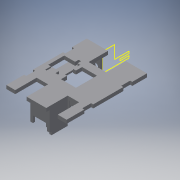
# Autodesk Inventor part: Fronthalf1
Saved by Autodesk Inventor 2016 (Build 200138000, 138)
## iProperties
Created: 2017-03-04
Part Number: Fronthalf1
Material: Generic
Document SubType Name: Modeling
Designer: Owner
Density: 1 g/cm^3
Appearance: Default
Author: Owner
Autodesk Inventor part; units mm, degrees
ref_plane "YZ Plane" through (0, 0, 0) normal (1, 0, 0) x (0, 1, 0)
ref_plane "XZ Plane" through (0, 0, 0) normal (0, 1, 0) x (-1, 0, 0)
ref_plane "XY Plane" through (0, 0, 0) normal (0, 0, 1) x (1, 0, 0)
sketch "Sketch1" plane through (0, 0, 0) normal (0, 1, 0) x (-1, 0, 0)
  line L0 (0, 0) -> (0, 114.3)
  line L1 (0, 114.3) -> (76.2, 114.3)
  line L2 (76.2, 114.3) -> (76.2, 0)
  line L3 (76.2, 0) -> (0, 0)
  circle A0 centre (38.1, 0) radius 38.1
  dimension "d0" = 114.3
  dimension "d1" = 76.2
  constraints: 8 end point, 2 perpendicular, 2 vertical, 1 horizontal alignment, 1 midpoint, 2 other
  measures "d0" distance of L0.start L0.end
  measures "d1" distance of L0.end L1.end
extrude "Extrusion1" add sketch "Sketch1" along normal blind 5
sketch "Sketch2" plane through (0, 0, 0) normal (0, -1, 0) x (1, 0, 0)
  line L0 (-27.94, 89.7) -> (-27.94, 77) projected
  line L1 (-48.26, 51.6) -> (-48.26, 64.3) projected
  line L2 (-48.26, 51.6) -> (-48.26, 49.6)
  line L3 (-53.34, 64.3) -> (-48.26, 64.3)
  line L4 (-48.26, 64.3) -> (-48.26, 66.3)
  line L5 (-27.94, 66.3) -> (-27.94, 49.6)
  line L6 (-48.26, 70.015) -> (-48.26, 45.885) projected
  line L7 (-48.26, 70.015) -> (-48.26, 45.885)
  line L8 (-48.26, 42.885) -> (-27.94, 42.885)
  line L9 (-27.94, 42.885) -> (-27.94, 72.015)
  line L10 (-27.94, 72.015) -> (-27.94, 73.015)
  line L11 (-27.94, 73.015) -> (-48.26, 73.015)
  line L12 (-48.26, 42.885) -> (-49.26, 42.885)
  line L13 (-49.0223, 73.0219) -> (-48.26, 73.015)
  line L14 (-27.94, 73.015) -> (-49.26, 73.015)
  line L15 (-49.26, 73.015) -> (-49.26, 42.885)
  line L16 (-49.26, 42.885) -> (-27.94, 42.885)
  line L17 (-27.94, 42.885) -> (-27.94, 73.015)
  point P0 (0, 0)
  dimension "d5" = 2
  dimension "d12" = 2
  dimension "d69" = 3
  dimension "d70" = 3
  dimension "d75" = 1
  constraints: 30 end point, 3 equal length, 3 horizontal, 3 perpendicular, 2 point on line, 2 vertical, 1 other
  measures "d5" distance of L1.start L2.end
  measures "d12" distance of L1.end L4.end
  measures "d69" distance of L6.start L11.end
  measures "d70" distance of L6.end L8.start
  measures "d75" distance of L8.start L12.end
extrude "Extrusion2" cut sketch "Sketch2" against normal blind 25.4
sketch "Sketch3" plane through (0, 0, 0) normal (0, -1, 0) x (1, 0, 0)
  arc A0 (-76.2, 0) -> (0, 0) centre (-38.1, 0) ccw projected
  line L0 (-38.1, 0) -> (-38.1, -27.5)
  circle A1 centre (-38.1, -27.5) radius 5
  dimension "d8" = 27.5
  dimension "d9" = 10
  constraints: 2 end point, 1 centre point, 1 coincident, 1 vertical
  measures "d8" distance of L0.start L0.end
  measures "d9" diameter of A1
extrude "Extrusion3" cut sketch "Sketch3" against normal blind 25.4
sketch "Sketch5" plane through (-76.2, 0, 114.3) normal (0, 0, 1) x (1, 0, 0)
  circle A0 centre (38.1, -23.375) radius 3.275 projected
  line L0 (47.85, -18.65) -> (28.35, -18.65) projected
  line L1 (28.35, -28.1) -> (47.85, -28.1) projected
  line L2 (28.35, -18.65) -> (28.35, -28.1) projected
  line L3 (47.85, -28.1) -> (47.85, -18.65) projected
  line L4 (76.2, 5) -> (0, 5) projected
  line L5 (38.1, 5) -> (38.1, -18.65)
  line L6 (38.1, -18.65) -> (47.85, -18.65)
  line L7 (47.85, -18.65) -> (48.1, -18.65)
  line L8 (48.1, -18.65) -> (48.1, -28.1)
  line L9 (48.1, -28.1) -> (52.1, -28.1)
  line L10 (52.1, -28.1) -> (52.1, -18.65)
  line L11 (52.1, -18.65) -> (52.1, -16.65)
  line L12 (52.1, -16.65) -> (52.1, 0)
  line L13 (0, 0) -> (76.2, 0) projected
  line L14 (38.1, -18.65) -> (28.35, -18.65)
  line L15 (28.35, -18.65) -> (28.1, -18.65)
  line L16 (28.1, -18.65) -> (28.1, -28.1)
  line L17 (28.1, -28.1) -> (24.1, -28.1)
  line L18 (24.1, -28.1) -> (24.1, 0)
  line L19 (52.1, 0) -> (24.1, 0)
  dimension "d23" = 0.25
  dimension "d24" = 4
  dimension "d25" = 2
  dimension "d26" = 0.25
  dimension "d27" = 4
  constraints: 28 end point, 9 point on line, 7 perpendicular, 2 midpoint, 1 collinear
  measures "d23" distance of L0.start L7.end
  measures "d24" distance of L8.end L9.end
  measures "d25" distance of L10.end L11.end
  measures "d26" distance of L0.end L15.end
  measures "d27" distance of L16.end L17.end
extrude "Extrusion5" add sketch "Sketch5" against normal blind 3 contours L0 L5 L13 L12 L11 L10 L9 L8 L7 | L0 L15 L16 L17 L18 L13 L5
ref_plane "Work Plane1" through (-76.2, 0, 79.55) normal (0, 0, -1) x (-1, 0, 0)
sketch "Sketch6" plane through (-76.2, 0, 79.55) normal (0, 0, -1) x (-1, 0, 0)
  circle A0 centre (-38.1, -23.375) radius 3.275 projected
  line L0 (-34.825, -23.375) -> (-30.825, -23.375)
  line L1 (-48.1, -18.65) -> (-28.1, -18.65) projected
  line L2 (-30.825, -23.375) -> (-30.825, 0)
  line L3 (-41.375, -23.375) -> (-45.375, -23.375)
  line L4 (0, 5) -> (-76.2, 5) projected
  line L5 (-45.375, -23.375) -> (-45.375, 0)
  line L6 (-45.375, 0) -> (-30.825, 0)
  circle A1 centre (-38.1, -23.375) radius 3.275
  point P0 (-76.2, 0)
  dimension "d31" = 4
  dimension "d32" = 4
  constraints: 10 end point, 3 perpendicular, 2 parallel, 2 point on circle, 1 centre point, 1 coincident, 1 concentric
  measures "d31" distance of L0.start L0.end
  measures "d32" distance of L3.start L3.end
extrude "Extrusion6" add sketch "Sketch6" along normal blind 3 contours A0 L3 L5 L1 L2 L0 | L1 L5 L6 L2
sketch "Sketch9" plane through (0, 0, 0) normal (0, -1, 0) x (1, 0, 0)
  line L0 (-45.375, 79.55) -> (-45.375, 76.55) projected
  line L1 (-44.442, 86.368) -> (-46.442, 86.368) projected
  line L2 (-46.442, 86.368) -> (-46.442, 79.796) projected
  line L3 (-46.442, 79.796) -> (-38.902, 79.796) projected
  line L4 (-38.902, 79.796) -> (-38.902, 86.368) projected
  line L5 (-38.902, 86.368) -> (-40.902, 86.368) projected
  line L6 (-40.902, 86.368) -> (-40.902, 81.796) projected
  line L7 (-40.902, 81.796) -> (-44.442, 81.796) projected
  line L8 (-44.442, 81.796) -> (-44.442, 86.368) projected
  line L9 (-41.375, 79.55) -> (-45.375, 79.55) projected
  line L10 (-45.375, 79.55) -> (-45.375, 76.55) projected
  line L11 (-41.375, 76.55) -> (-45.375, 76.55) projected
  line L12 (-41.375, 79.55) -> (-41.375, 76.55) projected
  line L13 (-45.375, 76.55) -> (-45.375, 79.55) projected
  line L14 (-46.442, 79.796) -> (-45.375, 79.796)
  line L15 (-45.375, 79.796) -> (-45.375, 76.55)
  line L16 (-45.375, 76.55) -> (-46.442, 76.55)
  line L17 (-46.442, 76.55) -> (-46.442, 79.796)
  line L18 (-38.902, 86.368) -> (-38.902, 79.796) projected
  line L19 (-38.902, 79.796) -> (-45.375, 79.796)
  line L20 (-45.375, 79.796) -> (-45.375, 79.55)
  line L21 (-45.375, 79.55) -> (-38.902, 79.55)
  line L22 (-38.902, 79.55) -> (-38.902, 79.796)
  point P0 (0, 0)
  constraints: 16 end point, 4 parallel, 2 horizontal, 2 perpendicular
extrude "Extrusion9" add sketch "Sketch9" along normal blind 23.37 contours L15 L3 L22 L21 L9 | L0 L16 L17 L3 L15
sketch "Sketch14" plane through (0, 0, 0) normal (0, -1, 0) x (1, 0, 0)
  line L0 (0, 0) -> (5, 0)
  line L1 (5, 0) -> (5, 114.3)
  line L2 (5, 114.3) -> (5, 119.3)
  line L3 (5, 119.3) -> (-76.2, 119.3)
  line L4 (-52.1, 114.3) -> (-76.2, 114.3) projected
  line L5 (-76.2, 119.3) -> (-81.2, 119.3)
  line L6 (-81.2, 119.3) -> (-81.2, 0)
  line L7 (-76.2, 0) -> (-81.2, 0)
  line L8 (-81.2, 0) -> (-81.2, 119.3)
  line L9 (-81.2, 119.3) -> (-76.2, 119.3)
  line L10 (-76.2, 119.3) -> (-76.2, 0)
  line L11 (-81.2, 119.3) -> (5, 119.3)
  line L12 (5, 119.3) -> (5, 114.3)
  line L13 (5, 114.3) -> (-81.2, 114.3)
  line L14 (-81.2, 114.3) -> (-81.2, 119.3)
  line L15 (5, 119.3) -> (0, 119.3)
  line L16 (0, 119.3) -> (0, 0)
  line L17 (0, 0) -> (5, 0)
  line L18 (5, 0) -> (5, 119.3)
  dimension "d58" = 5
  dimension "d59" = 5
  dimension "d60" = 5
  constraints: 36 end point, 7 parallel, 5 perpendicular, 4 horizontal, 3 point on line
  measures "d58" distance of L0.start L0.end
  measures "d59" distance of L1.end L2.end
  measures "d60" distance of L3.end L5.end
extrude "Extrusion14" add sketch "Sketch14" against normal blind 5
sketch "Sketch15" plane through (-38.902, -23.37, 79.55) normal (0, 0, -1) x (-1, 0, 0)
  arc A0 (2.473, -0.005) -> (-4.077, -0.005) centre (-0.802, -0.005) ccw projected
  circle A1 centre (-0.802, -0.005) radius 3.275
  point P0 (-38.902, 23.37)
  constraints: 1 centre point, 1 coincident
extrude "Extrusion15" cut sketch "Sketch15" against normal blind 25.4
ref_plane "Work Plane2" through (-29.1001, -34.45, 98.298) normal (1, 0, 0) x (0, -1, 0)
sketch "Sketch16" plane through (-29.1001, -34.45, 98.298) normal (1, 0, 0) x (0, -1, 0)
  line L0 (-5.08, 11.43) -> (5.08, 11.43) projected
  arc A0 (-5.08, 11.43) -> (-6.35, 10.16) centre (-5.08, 10.16) ccw projected
  line L1 (-6.35, -10.16) -> (-6.35, 10.16) projected
  arc A1 (-6.35, -10.16) -> (-5.08, -11.43) centre (-5.08, -10.16) ccw projected
  line L2 (5.08, -11.43) -> (-5.08, -11.43) projected
  arc A2 (5.08, -11.43) -> (6.35, -10.16) centre (5.08, -10.16) ccw projected
  line L3 (6.35, 10.16) -> (6.35, -10.16) projected
  arc A3 (6.35, 10.16) -> (5.08, 11.43) centre (5.08, 10.16) ccw projected
  line L4 (0, 11.43) -> (-6.35, 11.43)
  line L5 (-6.35, 11.43) -> (-6.35, -11.43)
  line L6 (-6.35, -11.43) -> (0, -11.43)
  line L7 (0, -11.43) -> (0, 11.43)
  line L8 (-34.45, -21.002) -> (-34.45, 98.298) projected
  line L9 (-6.35, 11.43) -> (-34.45, 11.43)
  line L10 (-34.45, 11.43) -> (-34.45, -11.43)
  line L11 (-34.45, -11.43) -> (-6.35, -11.43)
  line L12 (-6.35, -11.43) -> (-6.35, 11.43)
  constraints: 16 end point, 4 parallel, 2 horizontal, 2 perpendicular, 2 point on line, 1 midpoint
extrude "Extrusion16" add sketch "Sketch16" along normal blind 3 contours L0 L7 L2 A1 L1 A0 | A0 L5 L4 | L1 L5 L11 L8 L9 | A1 L6 L5
sketch "Sketch17" plane through (-29.1001, -34.45, 98.298) normal (-1, 0, 0) x (0, 0, 1)
  line L0 (10.16, 6.35) -> (-10.16, 6.35) projected
  line L1 (11.43, 34.45) -> (11.43, 0) projected
  line L2 (11.43, 34.45) -> (-11.43, 34.45) projected
  line L3 (11.43, 6.35) -> (-11.43, 6.35)
  line L4 (-11.43, 6.35) -> (-11.43, 34.45)
  line L5 (-11.43, 34.45) -> (11.43, 34.45)
  line L6 (11.43, 34.45) -> (11.43, 6.35)
  point P0 (-98.298, 34.45)
  constraints: 8 end point, 2 parallel, 1 horizontal, 1 perpendicular, 1 point on line
extrude "Extrusion17" add sketch "Sketch17" along normal blind 5
sketch "Sketch18" plane through (0, 0, 0) normal (0, -1, 0) x (1, 0, 0)
  line L0 (-76.2, 64.3) -> (-60.198, 64.3) projected
  line L1 (-70.866, 64.3) -> (-71.882, 64.3) projected
  line L2 (-70.866, 64.3) -> (-70.866, 66.84) projected
  line L3 (-71.882, 66.84) -> (-70.866, 66.84) projected
  line L4 (-76.2, 63.03) -> (-76.2, 64.3) projected
  line L5 (-76.2, 63.03) -> (-76.2, 42.71) projected
  line L6 (-76.2, 41.44) -> (-76.2, 42.71) projected
  line L7 (-76.2, 41.44) -> (-60.198, 41.44) projected
  line L8 (-60.198, 36.868) -> (-60.198, 42.71) projected
  line L9 (-57.658, 36.868) -> (-60.198, 36.868) projected
  line L10 (-57.658, 36.868) -> (-57.658, 42.71) projected
  line L11 (-57.658, 41.44) -> (-53.34, 41.44) projected
  line L12 (-53.34, 57.95) -> (-53.34, 42.71) projected
  line L13 (-53.34, 41.44) -> (-53.34, 42.71) projected
  line L14 (-53.34, 51.6) -> (-48.26, 51.6)
  line L15 (-53.34, 64.3) -> (-48.26, 64.3)
  line L16 (-57.658, 64.3) -> (-53.34, 64.3) projected
  line L17 (-57.658, 63.03) -> (-57.658, 68.872) projected
  line L18 (-60.198, 63.03) -> (-60.198, 68.872) projected
  line L19 (-57.658, 68.872) -> (-60.198, 68.872) projected
  line L20 (-48.26, 70.015) -> (-48.26, 45.885) projected
  line L21 (-76.2, 64.3) -> (-53.34, 64.3)
  line L22 (-53.34, 64.3) -> (-53.34, 41.44)
  line L23 (-53.34, 41.44) -> (-76.2, 41.44)
  line L24 (-76.2, 41.44) -> (-76.2, 64.3)
  line L25 (-57.658, 68.872) -> (-60.198, 68.872)
  line L26 (-60.198, 68.872) -> (-60.198, 64.3)
  line L27 (-60.198, 64.3) -> (-57.658, 64.3)
  line L28 (-57.658, 64.3) -> (-57.658, 68.872)
  line L29 (-60.198, 41.44) -> (-57.658, 41.44)
  line L30 (-57.658, 41.44) -> (-57.658, 36.868)
  line L31 (-57.658, 36.868) -> (-60.198, 36.868)
  line L32 (-60.198, 36.868) -> (-60.198, 41.44)
  line L33 (-71.882, 64.3) -> (-70.866, 64.3)
  line L34 (-70.866, 64.3) -> (-70.866, 66.84)
  line L35 (-53.34, 64.3) -> (-48.26, 64.3)
  line L36 (-48.26, 64.3) -> (-48.26, 51.6)
  line L37 (-48.26, 51.6) -> (-53.34, 51.6)
  line L38 (-53.34, 51.6) -> (-53.34, 64.3)
  line L39 (-70.866, 64.3) -> (-70.366, 64.3)
  line L40 (-70.366, 64.3) -> (-71.882, 64.3)
  line L41 (-71.882, 64.3) -> (-72.382, 64.3)
  line L42 (-70.366, 64.3) -> (-72.382, 64.3)
  line L43 (-72.382, 64.3) -> (-72.382, 72.555)
  line L44 (-72.382, 72.555) -> (-70.366, 72.555)
  line L45 (-70.366, 72.555) -> (-70.366, 64.3)
  line L46 (-60.698, 69.372) -> (-57.158, 69.372) projected
  line L47 (-60.698, 64.3) -> (-57.158, 64.3)
  line L48 (-57.158, 64.3) -> (-57.158, 69.372)
  line L49 (-57.158, 69.372) -> (-60.698, 69.372)
  line L50 (-60.698, 69.372) -> (-60.698, 64.3)
  line L51 (-60.698, 41.44) -> (-57.158, 41.44)
  line L52 (-57.158, 41.44) -> (-57.158, 36.368)
  line L53 (-57.158, 36.368) -> (-60.698, 36.368)
  line L54 (-60.698, 36.368) -> (-60.698, 41.44)
  point P0 (0, 0)
  dimension "d111" = 0.5
  dimension "d112" = 0.5
  dimension "d113" = 8.255
  constraints: 70 end point, 14 parallel, 10 horizontal, 8 perpendicular, 6 point on line, 1 collinear, 4 other
  measures "d111" distance of L33.end L39.end
  measures "d112" distance of L1.end L41.end
  measures "d113" distance of L42.end L43.end
extrude "Extrusion18" cut sketch "Sketch18" against normal blind 5
ref_plane "Work Plane3" through (-51.9601, -34.45, 98.306) normal (-1, 0, 0) x (0, -1, 0)
sketch "Sketch20" plane through (-51.9601, -34.45, 98.306) normal (-1, 0, 0) x (0, -1, 0)
  arc A0 (-6.35, 5.08) -> (6.35, 5.08) centre (0, 5.08) ccw projected
  line L0 (-6.35, 5.08) -> (-6.35, -10.16) projected
  arc A1 (-6.35, -10.16) -> (-5.08, -11.43) centre (-5.08, -10.16) ccw projected
  line L1 (-5.08, -11.43) -> (5.08, -11.43) projected
  arc A2 (5.08, -11.43) -> (6.35, -10.16) centre (5.08, -10.16) ccw projected
  line L2 (6.35, -10.16) -> (6.35, 5.08) projected
  line L3 (-6.35, -11.43) -> (-2.2139, -11.43)
  line L4 (-2.2139, -2.54) -> (-6.35, -2.54)
  line L5 (-6.35, -2.54) -> (-6.35, -11.43)
  line L6 (-6.35, -2.54) -> (-1.27, -2.54)
  line L7 (-1.27, -2.54) -> (-1.27, -11.43)
  line L8 (-6.35, -11.43) -> (-1.27, -11.43)
  line L9 (-1.27, -11.43) -> (-1.27, -2.54)
  line L10 (-1.27, -2.54) -> (-6.35, -2.54)
  line L11 (-6.35, -2.54) -> (-6.35, -11.43)
  point P0 (-34.45, -98.306)
  dimension "d76" = 8.89
  dimension "d77" = 4.1361
  dimension "d78" = 5.08
  constraints: 18 end point, 3 horizontal, 3 parallel, 2 perpendicular, 1 point on line
  measures "d76" distance of L3.end L4.start
  measures "d77" distance of L4.start L4.end
  measures "d78" distance of L4.end L6.end
extrude "Extrusion20" add sketch "Sketch20" along normal blind 2 contours L4 L6 L7 L1 A1 L0 | A1 L3 L5
sketch "Sketch21" plane through (-53.9601, -34.45, 98.306) normal (-1, 0, 0) x (0, 0, 1)
  line L0 (-2.54, 6.35) -> (-11.43, 6.35) projected
  line L1 (-11.438, 0) -> (-11.438, 34.45) projected
  line L2 (-2.54, 6.35) -> (-11.438, 6.35)
  line L3 (-11.438, 6.35) -> (-11.438, 34.45)
  line L4 (-11.438, 34.45) -> (-2.54, 34.45)
  line L5 (-2.54, 34.45) -> (-2.54, 6.35)
  point P0 (-98.306, 34.45)
  constraints: 8 end point, 2 parallel, 1 horizontal, 1 perpendicular
extrude "Extrusion21" add sketch "Sketch21" against normal blind 5
ref_plane "Work Plane4" through (-71.904, -22.7, 83.386) normal (0, 0, 1) x (-1, 0, 0)
ref_plane "Work Plane5" through (-43.18, -24.002, -27.5) normal (0, -1, 0) x (0, 0, -1)
sketch "Sketch23" plane through (-43.18, -24.002, -27.5) normal (0, -1, 0) x (0, 0, -1)
  circle A0 centre (0, 12.7) radius 1.016 projected
  arc A1 (-5.08, 11.43) -> (-6.35, 10.16) centre (-5.08, 10.16) ccw projected
  line L0 (5.08, 11.43) -> (-5.08, 11.43) projected
  arc A2 (6.35, 10.16) -> (5.08, 11.43) centre (5.08, 10.16) ccw projected
  line L1 (6.35, 10.16) -> (6.35, 16.002) projected
  line L2 (6.35, 16.002) -> (-6.35, 16.002) projected
  line L3 (-6.35, 16.002) -> (-6.35, 10.16) projected
  arc A3 (-6.35, -10.16) -> (-5.08, -11.43) centre (-5.08, -10.16) ccw projected
  line L4 (-6.35, -10.16) -> (-6.35, -16.002) projected
  line L5 (-6.35, -16.002) -> (6.35, -16.002) projected
  line L6 (6.35, -16.002) -> (6.35, -10.16) projected
  arc A4 (5.08, -11.43) -> (6.35, -10.16) centre (5.08, -10.16) ccw projected
  line L7 (-5.08, -11.43) -> (5.08, -11.43) projected
  circle A5 centre (0, -12.7) radius 1.016 projected
  line L8 (6.35, 11.43) -> (-6.35, 11.43)
  line L9 (-6.35, 11.43) -> (-6.35, 16.002)
  line L10 (-6.35, 16.002) -> (6.35, 16.002)
  line L11 (6.35, 16.002) -> (6.35, 11.43)
  circle A6 centre (0, 12.7) radius 1.016
  line L12 (-6.35, -11.43) -> (6.35, -11.43)
  line L13 (6.35, -11.43) -> (6.35, -16.002)
  line L14 (6.35, -16.002) -> (-6.35, -16.002)
  line L15 (-6.35, -16.002) -> (-6.35, -11.43)
  circle A7 centre (0, -12.7) radius 1.016
  line L16 (6.35, 11.43) -> (-31.75, 11.43)
  line L17 (-31.75, 11.43) -> (-31.75, 16.002)
  line L18 (-31.75, 16.002) -> (6.35, 16.002)
  line L19 (6.35, 16.002) -> (6.35, 11.43)
  line L20 (6.35, -16.002) -> (-31.75, -16.002)
  line L21 (-31.75, -16.002) -> (-31.75, -11.43)
  line L22 (-31.75, -11.43) -> (6.35, -11.43)
  line L23 (6.35, -11.43) -> (6.35, -16.002)
  point P0 (-27.5, 43.18)
  dimension "d89" = 38.1
  dimension "d90" = 38.1
  constraints: 32 end point, 8 parallel, 4 horizontal, 4 perpendicular, 2 centre point, 2 coincident, 2 concentric, 2 point on line
  measures "d89" distance of L17.end L18.end
  measures "d90" distance of L5.end L20.end
extrude "Extrusion23" add sketch "Sketch23" along normal blind 3 contours L8 L3 L2 L1 L0 | L16 L17 L18 L3 | L7 L12 L6 L5 L4 | L4 L20 L21 L22
sketch "Sketch24" plane through (-59.182, -24.002, -33.85) normal (-1, 0, 0) x (0, 0, 1)
  line L0 (38.1, 0) -> (38.1, -3) projected
  line L1 (-4.25, 24.002) -> (33.85, 24.002) projected
  line L2 (38.1, -3) -> (20.32, -3)
  line L3 (20.32, -3) -> (20.32, 24.002)
  line L4 (20.32, 24.002) -> (38.1, 24.002)
  line L5 (38.1, 24.002) -> (38.1, -3)
  dimension "d93" = 17.78
  constraints: 8 end point, 2 parallel, 1 horizontal, 1 perpendicular, 1 point on line
  measures "d93" distance of L0.end L2.end
extrude "Extrusion24" add sketch "Sketch24" against normal blind 32.004
ref_plane "Work Plane6" through (-43.18, -21.462, -27.5) normal (0, 1, 0) x (0, 0, 1)
sketch "Sketch25" plane through (-43.18, -21.462, -27.5) normal (0, 1, 0) x (0, 0, 1)
  arc A0 (5.08, -11.43) -> (6.35, -10.16) centre (5.08, -10.16) ccw projected
  line L0 (-5.08, -11.43) -> (5.08, -11.43) projected
  arc A1 (-6.35, -10.16) -> (-5.08, -11.43) centre (-5.08, -10.16) ccw projected
  line L1 (-6.35, -16.002) -> (-6.35, -10.16) projected
  line L2 (6.35, -16.002) -> (-6.35, -16.002) projected
  line L3 (6.35, -10.16) -> (6.35, -16.002) projected
  circle A2 centre (0, -12.7) radius 1.016 projected
  arc A3 (6.35, 10.16) -> (5.08, 11.43) centre (5.08, 10.16) ccw projected
  line L4 (6.35, 16.002) -> (6.35, 10.16) projected
  line L5 (-6.35, 16.002) -> (6.35, 16.002) projected
  line L6 (-6.35, 10.16) -> (-6.35, 16.002) projected
  arc A4 (-5.08, 11.43) -> (-6.35, 10.16) centre (-5.08, 10.16) ccw projected
  line L7 (5.08, 11.43) -> (-5.08, 11.43) projected
  circle A5 centre (0, 12.7) radius 1.016 projected
  line L8 (31.75, 16.002) -> (13.97, 16.002) projected
  line L9 (-6.35, 11.43) -> (22.86, 11.43)
  line L10 (22.86, 11.43) -> (22.86, 16.002)
  line L11 (22.86, 16.002) -> (-6.35, 16.002)
  line L12 (-6.35, 16.002) -> (-6.35, 11.43)
  circle A6 centre (0, 12.7) radius 1.016
  line L13 (-6.35, -11.43) -> (13.97, -11.43)
  line L14 (13.97, -11.43) -> (13.97, -16.002)
  line L15 (13.97, -16.002) -> (-6.35, -16.002)
  line L16 (-6.35, -16.002) -> (-6.35, -11.43)
  circle A7 centre (0, -12.7) radius 1.016
  point P0 (27.5, 43.18)
  constraints: 16 end point, 4 parallel, 2 centre point, 2 coincident, 2 concentric, 2 horizontal, 2 perpendicular, 2 point on line, 1 midpoint
extrude "Extrusion25" add sketch "Sketch25" along normal blind 3 contours L13 L3 L2 L1 L0 | L13 L14 L15 L3 | L7 L9 L6 L5 L4 | L4 L11 L8 L10 L9
sketch "Sketch26" plane through (-43.18, -21.462, -27.5) normal (0, -1, 0) x (1, 0, 0)
  line L0 (16.002, 6.35) -> (10.16, 6.35) projected
  line L1 (-16.002, -6.35) -> (-16.002, 13.97) projected
  line L2 (-16.002, 13.97) -> (-11.43, 13.97) projected
  line L3 (-16.002, 6.35) -> (-13.716, 6.35)
  line L4 (-13.716, 6.35) -> (-13.716, 13.97)
  line L5 (-13.716, 13.97) -> (-16.002, 13.97)
  line L6 (-16.002, 13.97) -> (-16.002, 6.35)
  line L7 (-13.716, 13.97) -> (-11.8721, 13.97)
  line L8 (-11.8721, 13.97) -> (-11.8721, 6.35)
  line L9 (-11.8721, 6.35) -> (-13.716, 6.35)
  line L10 (-13.716, 6.35) -> (-13.716, 13.97)
  line L11 (11.43, 13.97) -> (16.002, 13.97) projected
  line L12 (11.43, 6.35) -> (16.002, 6.35)
  line L13 (16.002, 6.35) -> (16.002, 13.97)
  line L14 (16.002, 13.97) -> (11.43, 13.97)
  line L15 (11.43, 13.97) -> (11.43, 6.35)
  point P0 (43.18, 27.5)
  constraints: 24 end point, 6 parallel, 3 horizontal, 3 perpendicular, 2 point on line, 1 midpoint
extrude "Extrusion26" add sketch "Sketch26" along normal blind 3
sketch "Sketch28" plane through (0, 0, 0) normal (0, -1, 0) x (1, 0, 0)
  line L0 (-81.2, 119.3) -> (-81.2, 93.9)
  line L1 (-81.2, 119.3) -> (-81.2, 0) projected
  line L2 (-81.2, 93.9) -> (-78.2, 93.9)
  line L3 (-78.2, 93.9) -> (-78.2, 81.2)
  line L4 (-78.2, 81.2) -> (-81.2, 81.2)
  line L5 (-81.2, 93.9) -> (-81.2, 81.2)
  line L6 (-81.2, 0) -> (-76.2, 0) projected
  line L7 (-81.2, 0) -> (-81.2, 25.4)
  line L8 (-81.2, 25.4) -> (-78.2, 25.4)
  line L9 (-78.2, 25.4) -> (-78.2, 38.1)
  line L10 (-78.2, 38.1) -> (-81.2, 38.1)
  line L11 (-81.2, 25.4) -> (-81.2, 38.1)
  line L12 (5, 119.3) -> (-81.2, 119.3) projected
  line L13 (-38.1, 119.3) -> (-38.1, 128.3765)
  line L14 (5, 119.3) -> (5, 93.9)
  line L15 (5, 119.3) -> (5, 0)
  line L16 (5, 93.9) -> (2, 93.9)
  line L17 (2, 93.9) -> (2, 81.2)
  line L18 (2, 81.2) -> (5, 81.2)
  line L19 (5, 93.9) -> (5, 81.2)
  line L20 (5, 0) -> (5, 25.4)
  line L21 (5, 25.4) -> (2, 25.4)
  line L22 (2, 25.4) -> (2, 38.1)
  line L23 (2, 38.1) -> (5, 38.1)
  line L24 (5, 25.4) -> (5, 38.1)
  point P0 (0, 0)
  dimension "d104" = 25.4
  dimension "d105" = 3
  dimension "d106" = 12.7
  dimension "d107" = 25.4
  dimension "d108" = 12.7
  constraints: 44 end point, 12 point on line, 9 symmetric about line, 5 perpendicular, 2 collinear, 1 midpoint, 1 vertical
  measures "d104" distance of L0.start L0.end
  measures "d105" distance of L0.end L2.end
  measures "d106" distance of L2.end L3.end
  measures "d107" distance of L1.end L7.end
  measures "d108" distance of L8.end L9.end
extrude "Extrusion27" cut sketch "Sketch28" against normal blind 254
sketch "Sketch29" plane through (0, 5, 0) normal (0, 1, 0) x (1, 0, 0)
  circle A0 centre (-38.1, 27.5) radius 5 projected
  circle A1 centre (-38.1, 27.5) radius 5
  point P0 (0, 0)
  constraints: 1 centre point, 1 coincident
extrude "Extrusion28" add sketch "Sketch29" against normal blind 5.0038
sketch "Sketch30" plane through (0, 0, 0) normal (0, -1, 0) x (1, 0, 0)
  line L0 (-25.7555, 33.65) -> (-0.7555, 33.65) projected
  line L1 (-0.7555, 33.65) -> (-0.7555, 85.65) projected
  line L2 (-0.7555, 85.65) -> (-25.7555, 85.65) projected
  line L3 (-25.7555, 85.65) -> (-25.7555, 33.65) projected
  line L4 (-27.94, 42.885) -> (-25.7555, 42.885)
  line L5 (-25.7555, 42.885) -> (-25.7555, 69.015)
  line L6 (-25.7555, 69.015) -> (-27.94, 69.015)
  line L7 (-27.94, 69.015) -> (-27.94, 42.885)
  line L8 (-25.7555, 85.65) -> (-20.7555, 85.65)
  line L9 (-0.7555, 85.65) -> (-5.7555, 85.65)
  line L10 (-20.7555, 85.65) -> (-5.7555, 85.65)
  line L11 (-5.7555, 85.65) -> (-5.7555, 88.65)
  line L12 (-5.7555, 88.65) -> (-20.7555, 88.65)
  line L13 (-20.7555, 88.65) -> (-20.7555, 85.65)
  point P0 (0, 0)
  dimension "d116" = 5
  dimension "d117" = 5
  dimension "d118" = 3
  constraints: 20 end point, 4 parallel, 3 point on line, 2 horizontal, 2 perpendicular
  measures "d116" distance of L2.end L8.end
  measures "d117" distance of L1.end L9.end
  measures "d118" distance of L10.end L11.end
extrude "Extrusion29" add sketch "Sketch30" along normal blind 5 contours L4 L7 L6 L3 | L2 L13 L12 L11
sketch "Sketch31" plane through (-24.1, -28.1, 114.3) normal (1, 0, 0) x (0, 0, -1)
  line L0 (0, 0) -> (0, 9.45) projected
  line L1 (4.572, 28.1) -> (4.572, -6.35) projected
  line L2 (0, 0) -> (4.572, 0)
  line L3 (4.572, 0) -> (4.572, 28.1)
  line L4 (4.572, 28.1) -> (0, 28.1)
  line L5 (0, 28.1) -> (0, 0)
  point P0 (114.3, 28.1)
  constraints: 8 end point, 2 parallel, 1 horizontal, 1 perpendicular
extrude "Extrusion30" add sketch "Sketch31" against normal blind 4
sketch "Sketch32" plane through (0, 0, 0) normal (0, -1, 0) x (1, 0, 0)
  line L0 (-57.158, 69.372) -> (-57.158, 64.3) projected
  line L1 (-57.158, 69.372) -> (-70.366, 69.372)
  line L2 (-70.366, 69.372) -> (-70.366, 36.368)
  line L3 (-70.366, 36.368) -> (-57.158, 36.368)
  line L4 (-57.158, 36.368) -> (-57.158, 69.372)
  point P0 (0, 0)
  constraints: 8 end point, 2 parallel, 1 horizontal, 1 perpendicular
extrude "Extrusion31" add sketch "Sketch32" along normal blind 2.54
sketch "Sketch35" plane through (-59.182, -27.002, 4.25) normal (0, 0, 1) x (1, 0, 0)
  circle A0 centre (21.082, 3.627) radius 1.9 projected
  circle A1 centre (21.082, 3.627) radius 1.9
  circle A2 centre (21.082, 3.627) radius 1.9
  line L0 (32.004, 0) -> (0, 0) projected
  line L1 (22.982, 0) -> (19.182, 0)
  line L2 (22.982, 0) -> (21.082, 0)
  line L3 (21.082, 0) -> (21.082, 3.627)
  line L4 (21.082, 3.627) -> (22.982, 3.627)
  line L5 (22.982, 3.627) -> (22.982, 0)
  line L6 (21.082, 3.627) -> (19.182, 3.627)
  line L7 (19.182, 3.627) -> (19.182, 0)
  line L8 (19.182, 0) -> (21.082, 0)
  line L9 (21.082, 0) -> (21.082, 3.627)
  point P0 (59.182, 27.002)
  constraints: 18 end point, 4 parallel, 2 centre point, 2 coincident, 2 horizontal, 2 perpendicular, 2 point on line, 1 concentric
extrude "Extrusion34" cut sketch "Sketch35" against normal blind 25.4
sketch "Sketch36" plane through (0, 5, 0) normal (0, 1, 0) x (1, 0, 0)
  line L0 (-81.2, -119.3) -> (5, -119.3) projected
  line L1 (-81.2, -119.3) -> (-68.5, -119.3)
  line L2 (5, -119.3) -> (-7.7, -119.3)
  line L3 (-5.7555, -88.65) -> (-20.7555, -88.65) projected
  line L4 (-68.5, -119.3) -> (-7.7, -119.3)
  line L5 (-7.7, -119.3) -> (-7.7, -88.65)
  line L6 (-7.7, -88.65) -> (-68.5, -88.65)
  line L7 (-68.5, -88.65) -> (-68.5, -119.3)
  line L8 (-52.1, -111.3) -> (-52.1, -114.3) projected
  line L9 (-24.1, -114.3) -> (-24.1, -109.728) projected
  line L10 (-52.1, -119.3) -> (-68.5, -119.3)
  line L11 (-68.5, -119.3) -> (-68.5, -88.65)
  line L12 (-68.5, -88.65) -> (-52.1, -88.65)
  line L13 (-52.1, -88.65) -> (-52.1, -119.3)
  line L14 (-24.1, -119.3) -> (-7.7, -119.3)
  line L15 (-7.7, -119.3) -> (-7.7, -88.65)
  line L16 (-7.7, -88.65) -> (-24.1, -88.65)
  line L17 (-24.1, -88.65) -> (-24.1, -119.3)
  point P0 (0, 0)
  dimension "d134" = 12.7
  dimension "d135" = 12.7
  constraints: 28 end point, 6 parallel, 5 point on line, 3 horizontal, 3 perpendicular
  measures "d134" distance of L0.start L1.end
  measures "d135" distance of L0.end L2.end
sketch "Sketch37" plane through (0, 0, 0) normal (0, -1, 0) x (1, 0, 0)
  line L0 (-29.1001, 88.146) -> (-45.1021, 88.146) projected
  line L1 (-29.1001, 88.146) -> (-29.1001, 108.466) projected
  line L2 (-29.1001, 108.466) -> (-45.1021, 108.466) projected
  line L3 (-45.1021, 114.308) -> (-45.1021, 108.466) projected
  line L4 (-47.6421, 114.308) -> (-45.1021, 114.308) projected
  line L5 (-47.6421, 114.308) -> (-47.6421, 108.466) projected
  line L6 (-47.6421, 108.466) -> (-51.9601, 108.466) projected
  line L7 (-51.9601, 103.386) -> (-51.9601, 108.466) projected
  line L8 (-51.9601, 88.146) -> (-51.9601, 103.386) projected
  line L9 (-47.6421, 88.146) -> (-51.9601, 88.146) projected
  line L10 (-47.6421, 88.146) -> (-47.6421, 82.304) projected
  line L11 (-47.6421, 82.304) -> (-45.1021, 82.304) projected
  line L12 (-45.1021, 88.146) -> (-45.1021, 82.304) projected
  line L13 (-47.6421, 82.304) -> (-47.7421, 82.304)
  line L14 (-47.7421, 82.304) -> (-47.7421, 82.204)
  line L15 (-47.7421, 82.204) -> (-47.7421, 84.704)
  line L16 (-47.7421, 84.704) -> (-50.2421, 84.704)
  line L17 (-47.7421, 82.204) -> (-45.1021, 82.204)
  line L18 (-45.1021, 82.204) -> (-45.0021, 82.204)
  line L19 (-45.0021, 82.204) -> (-45.0021, 84.704)
  line L20 (-45.0021, 84.704) -> (-42.5021, 84.704)
  line L21 (-42.5021, 84.704) -> (-42.5021, 79.796)
  line L22 (-46.442, 79.796) -> (-38.902, 79.796) projected
  line L23 (-50.2421, 84.704) -> (-50.2421, 79.796)
  line L24 (-50.2421, 79.796) -> (-46.442, 79.796)
  point P0 (0, 0)
  dimension "d136" = 0.1
  dimension "d137" = 0.1
  dimension "d138" = 2.5
  dimension "d139" = 2.5
  dimension "d140" = 0.1
  dimension "d141" = 2.5
  constraints: 22 end point, 6 perpendicular, 2 horizontal, 2 point on line, 2 vertical
  measures "d136" distance of L10.end L13.end
  measures "d137" distance of L13.end L14.end
  measures "d138" distance of L14.end L15.end
  measures "d139" distance of L15.end L16.end
  measures "d140" distance of L17.end L18.end
  measures "d141" distance of L19.end L20.end
extrude "Extrusion35" add sketch "Sketch37" along normal blind 40.894 contours L14 L17 L18 L19 L20 L21 L22 L24 L23 L16 L15
extrude "Extrusion36" cut sketch "Sketch36" against normal blind 5.08 contours L7 L6 L13 L8 L0 | L17 L9 L6 L3 L5 L0
sketch "Sketch38" plane through (0, -2.54, 0) normal (0, -1, 0) x (1, 0, 0)
  line L0 (-73.7193, 68.8881) -> (-54.2193, 68.8881) projected
  line L1 (-57.158, 64.3) -> (-57.158, 69.372) projected
  line L2 (-70.366, 64.3) -> (-70.366, 41.44) projected
  line L3 (-57.158, 68.8881) -> (-70.366, 68.8881)
  line L4 (-70.366, 68.8881) -> (-70.366, 65.8881)
  line L5 (-70.366, 65.8881) -> (-57.158, 65.8881)
  line L6 (-57.158, 65.8881) -> (-57.158, 68.8881)
  point P0 (0, 0)
  dimension "d146" = 3
  constraints: 8 end point, 3 point on line, 2 parallel, 1 horizontal, 1 perpendicular
  measures "d146" distance between parallel lines of L5 L0
extrude "Extrusion37" add sketch "Sketch38" along normal blind 21.59
sketch "Sketch39" plane through (0, 0, 0) normal (0, -1, 0) x (1, 0, 0)
  line L0 (-67.2443, -4.7119) -> (-60.6943, -4.7119) projected
  line L1 (-70.366, 36.368) -> (-70.366, 41.44) projected
  line L2 (-70.366, 36.368) -> (-70.366, 5.888)
  line L3 (-70.366, 5.888) -> (-57.158, 5.888)
  line L4 (-70.366, 5.888) -> (-57.158, 5.888)
  line L5 (-57.158, 5.888) -> (-57.158, 8.888)
  line L6 (-57.158, 8.888) -> (-70.366, 8.888)
  line L7 (-70.366, 8.888) -> (-70.366, 5.888)
  point P0 (0, 0)
  dimension "d149" = 30.48
  dimension "d150" = 3
  constraints: 12 end point, 2 parallel, 2 perpendicular, 1 horizontal, 1 vertical
  measures "d149" distance of L1.start L2.end
  measures "d150" distance of L4.end L5.end
extrude "Extrusion38" add sketch "Sketch39" along normal blind 27.94
sketch "Sketch40" plane through (-57.158, 0, 5.888) normal (0, 0, -1) x (-1, 0, 0)
  circle A0 centre (6.8113, -17.72) radius 3.275 projected
  circle A1 centre (6.8113, -17.72) radius 3.556
  point P0 (-57.158, 0)
  dimension "d153" = 7.112
  constraints: 1 centre point, 1 coincident
  measures "d153" diameter of A1
extrude "Extrusion39" cut sketch "Sketch40" against normal blind 76.2 contours A0 | A1
sketch "Sketch41" plane through (-59.182, -27.002, 4.25) normal (-1, 0, 0) x (0, 0, 1)
  line L0 (-25.4, 3) -> (-38.1, 3) projected
  line L1 (-38.1, 3) -> (-38.1, 0) projected
  line L2 (0, 0) -> (-38.1, 0) projected
  line L3 (0, 27.002) -> (0, 0) projected
  line L4 (-17.78, 27.002) -> (0, 27.002) projected
  line L5 (-17.78, 8.54) -> (-17.78, 27.002) projected
  line L6 (-38.1, 8.54) -> (-17.78, 8.54) projected
  line L7 (-38.1, 5.54) -> (-38.1, 8.54) projected
  line L8 (-38.1, 5.54) -> (-25.4, 5.54) projected
  line L9 (-25.4, 5.54) -> (-25.4, 3) projected
  point P0 (-4.25, 27.002)
sketch "Sketch42" plane through (0, 0, 0) normal (0, -1, 0) x (1, 0, 0)
  line L0 (-70.366, 5.888) -> (-70.366, 8.888) projected
  line L1 (-70.366, 8.888) -> (-57.158, 8.888) projected
  line L2 (-57.158, 8.888) -> (-57.158, 5.888) projected
  line L3 (-57.158, 5.888) -> (-70.366, 5.888) projected
  line L4 (-24.1, 88.65) -> (-24.1, 109.728) projected
  line L5 (-24.1, 109.728) -> (-26.1001, 109.728) projected
  line L6 (-26.1001, 109.728) -> (-26.1001, 86.868) projected
  line L7 (-26.1001, 86.868) -> (-34.1001, 86.868) projected
  line L8 (-34.1001, 86.868) -> (-34.1001, 109.728) projected
  line L9 (-34.1001, 109.728) -> (-28.1, 109.728) projected
  line L10 (-28.1, 109.728) -> (-28.1, 111.3) projected
  line L11 (-28.1, 111.3) -> (-52.1, 111.3) projected
  line L12 (-52.1, 111.3) -> (-52.1, 95.766) projected
  line L13 (-52.1, 95.766) -> (-48.9601, 95.766) projected
  line L14 (-48.9601, 95.766) -> (-48.9601, 86.868) projected
  line L15 (-48.9601, 86.868) -> (-53.9601, 86.868) projected
  line L16 (-53.9601, 86.868) -> (-53.9601, 88.65) projected
  line L17 (-53.9601, 88.65) -> (-68.5, 88.65) projected
  line L18 (-68.5, 88.65) -> (-68.5, 119.3) projected
  line L19 (-68.5, 119.3) -> (-81.2, 119.3) projected
  line L20 (-81.2, 119.3) -> (-81.2, 93.9) projected
  line L21 (-81.2, 93.9) -> (-78.2, 93.9) projected
  line L22 (-78.2, 93.9) -> (-78.2, 81.2) projected
  line L23 (-78.2, 81.2) -> (-81.2, 81.2) projected
  line L24 (-81.2, 81.2) -> (-81.2, 38.1) projected
  line L25 (-81.2, 38.1) -> (-78.2, 38.1) projected
  line L26 (-78.2, 38.1) -> (-78.2, 25.4) projected
  line L27 (-78.2, 25.4) -> (-81.2, 25.4) projected
  line L28 (-81.2, 25.4) -> (-81.2, 0) projected
  line L29 (-81.2, 0) -> (-76.2, 0) projected
  arc A0 (-76.2, 0) -> (0, 0) centre (-38.1, 0) ccw projected
  line L30 (0, 0) -> (5, 0) projected
  line L31 (5, 0) -> (5, 25.4) projected
  line L32 (5, 25.4) -> (2, 25.4) projected
  line L33 (2, 25.4) -> (2, 38.1) projected
  line L34 (2, 38.1) -> (5, 38.1) projected
  line L35 (5, 38.1) -> (5, 81.2) projected
  line L36 (5, 81.2) -> (2, 81.2) projected
  line L37 (2, 81.2) -> (2, 93.9) projected
  line L38 (2, 93.9) -> (5, 93.9) projected
  line L39 (5, 93.9) -> (5, 119.3) projected
  line L40 (5, 119.3) -> (-7.7, 119.3) projected
  line L41 (-7.7, 119.3) -> (-7.7, 88.65) projected
  line L42 (-7.7, 88.65) -> (-5.7555, 88.65) projected
  line L43 (-5.7555, 88.65) -> (-5.7555, 85.65) projected
  line L44 (-5.7555, 85.65) -> (-20.7555, 85.65) projected
  line L45 (-20.7555, 85.65) -> (-20.7555, 88.65) projected
  line L46 (-20.7555, 88.65) -> (-24.1, 88.65) projected
  line L47 (-27.178, -13.53) -> (-59.182, -13.53) projected
  line L48 (-59.182, -13.53) -> (-59.182, 4.25) projected
  line L49 (-59.182, 4.25) -> (-27.178, 4.25) projected
  line L50 (-27.178, 4.25) -> (-27.178, -13.53) projected
  line L51 (-46.442, 79.796) -> (-50.2421, 79.796) projected
  line L52 (-50.2421, 79.796) -> (-50.2421, 84.704) projected
  line L53 (-50.2421, 84.704) -> (-47.7421, 84.704) projected
  line L54 (-47.7421, 84.704) -> (-47.7421, 82.204) projected
  line L55 (-47.7421, 82.204) -> (-45.0021, 82.204) projected
  line L56 (-45.0021, 82.204) -> (-45.0021, 84.704) projected
  line L57 (-45.0021, 84.704) -> (-42.5021, 84.704) projected
  line L58 (-42.5021, 84.704) -> (-42.5021, 79.796) projected
  line L59 (-42.5021, 79.796) -> (-38.902, 79.796) projected
  line L60 (-38.902, 79.796) -> (-38.902, 79.55) projected
  line L61 (-38.902, 79.55) -> (-30.825, 79.55) projected
  line L62 (-30.825, 79.55) -> (-30.825, 76.55) projected
  line L63 (-30.825, 76.55) -> (-46.442, 76.55) projected
  line L64 (-46.442, 76.55) -> (-46.442, 79.796) projected
  circle A1 centre (-38.1, -27.5) radius 5 projected
  line L65 (-70.366, 36.368) -> (-70.366, 41.44) projected
  line L66 (-70.366, 41.44) -> (-76.2, 41.44) projected
  line L67 (-76.2, 41.44) -> (-76.2, 64.3) projected
  line L68 (-76.2, 64.3) -> (-72.382, 64.3) projected
  line L69 (-72.382, 64.3) -> (-72.382, 72.555) projected
  line L70 (-72.382, 72.555) -> (-70.366, 72.555) projected
  line L71 (-70.366, 72.555) -> (-70.366, 69.372) projected
  line L72 (-70.366, 69.372) -> (-60.698, 69.372) projected
  line L73 (-60.698, 69.372) -> (-57.158, 69.372) projected
  line L74 (-57.158, 69.372) -> (-57.158, 64.3) projected
  line L75 (-57.158, 64.3) -> (-49.26, 64.3) projected
  line L76 (-49.26, 64.3) -> (-49.26, 73.015) projected
  line L77 (-49.26, 73.015) -> (-27.94, 73.015) projected
  line L78 (-27.94, 73.015) -> (-27.94, 69.015) projected
  line L79 (-27.94, 69.015) -> (-25.7555, 69.015) projected
  line L80 (-25.7555, 69.015) -> (-25.7555, 42.885) projected
  line L81 (-25.7555, 42.885) -> (-27.94, 42.885) projected
  line L82 (-27.94, 42.885) -> (-49.26, 42.885) projected
  line L83 (-49.26, 42.885) -> (-49.26, 51.6) projected
  line L84 (-49.26, 51.6) -> (-53.34, 51.6) projected
  line L85 (-53.34, 51.6) -> (-53.34, 41.44) projected
  line L86 (-53.34, 41.44) -> (-57.158, 41.44) projected
  line L87 (-57.158, 41.44) -> (-57.158, 36.368) projected
  line L88 (-57.158, 36.368) -> (-60.698, 36.368) projected
  line L89 (-60.698, 36.368) -> (-70.366, 36.368) projected
  line L90 (5, 4.25) -> (-81.2, 4.25)
  line L91 (-81.2, 4.25) -> (-81.2, -51.7211)
  line L92 (-81.2, -51.7211) -> (5, -51.7211)
  line L93 (5, -51.7211) -> (5, 4.25)
  constraints: 8 end point, 2 parallel, 1 horizontal, 1 perpendicular, 1 point on line
extrude "Extrusion40" cut sketch "Sketch42" along normal mid plane 25120.6 contours L31 L30 A0 L29 L28 L90 L48 L47 L50 | L93 L92 L91 L29 A0 L30 | L50 L47 L48 L49 | A1
sketch "Sketch43" plane through (0, 5, 0) normal (0, 1, 0) x (1, 0, 0)
  line L0 (-81.2, -4.25) -> (-50.8, -4.25) projected
  line L1 (-50.8, -4.25) -> (-50.8, -31.75) projected
  line L2 (-50.8, -31.75) -> (-25.4, -31.75) projected
  line L3 (-25.4, -31.75) -> (-25.4, -4.25) projected
  line L4 (-25.4, -4.25) -> (5, -4.25) projected
  line L5 (5, -4.25) -> (5, 0) projected
  line L6 (5, 0) -> (0, 0) projected
  arc A0 (0, 0) -> (-76.2, 0) centre (-38.1, 0) ccw projected
  line L7 (-76.2, 0) -> (-81.2, 0) projected
  line L8 (-81.2, 0) -> (-81.2, -4.25) projected
  line L9 (-50.8, -31.75) -> (-51.05, -31.75)
  line L10 (-51.05, -31.75) -> (-51.05, -32)
  line L11 (-25.4, -4.25) -> (-25.15, -4.25)
  line L12 (5, -4.25) -> (-81.2, -4.25) projected
  line L13 (-25.15, -4.25) -> (-51.05, -4.25)
  line L14 (-51.05, -4.25) -> (-51.05, -32)
  line L15 (-51.05, -32) -> (-25.15, -32)
  line L16 (-25.15, -32) -> (-25.15, -4.25)
  dimension "d158" = 0.25
  dimension "d159" = 0.25
  dimension "d160" = 0.25
  constraints: 14 end point, 2 horizontal, 2 parallel, 2 perpendicular, 1 point on line
  measures "d158" distance of L1.end L9.end
  measures "d159" distance of L9.end L10.end
  measures "d160" distance of L3.end L11.end
extrude "Extrusion41" cut sketch "Sketch43" against normal blind 25.4 contours L12 L3 L2 L1 | L9 L2 L3 L4 L16 L15 L10
body "Solid1"
